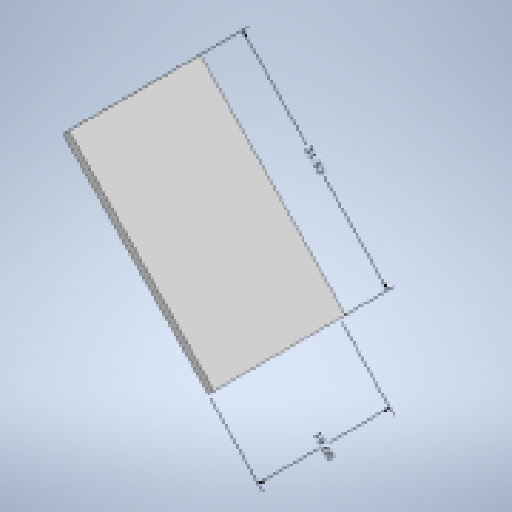
# Autodesk Inventor part: BarraInclinada
Saved by Autodesk Inventor 2024 (Build 280153000, 153)
## iProperties
Created: 2023-07-05
Part Number: BarraInclinada
Material: Genérico
Document SubType Name: Modeling
Designer: sergi
Density: 1 g/cm^3
Appearance: Valor por defecto
Author: sergi
Autodesk Inventor part; units mm, degrees
ref_plane "YZ Plane" through (0, 0, 0) normal (1, 0, 0) x (0, 1, 0)
ref_plane "XZ Plane" through (0, 0, 0) normal (0, 1, 0) x (-1, 0, 0)
ref_plane "XY Plane" through (0, 0, 0) normal (0, 0, 1) x (1, 0, 0)
ref_plane "Plano de trabajo1" through (-734, 252.5, -55) normal (0, 0, -1) x (0, -1, 0)
ref_plane "Plano de trabajo2" through (-30, -30, 770) normal (-1, 0, 0) x (0, 1, 0)
sketch "Boceto4" plane through (-30, -30, 770) normal (-1, 0, 0) x (0, 1, 0)
  line L0 (30, 770) -> (551, 770) projected
  line L1 (1956, 770) -> (581, 770) projected
  line L2 (611, 770) -> (581, 770) projected
  line L3 (30, 770) -> (596, 770)
  line L4 (596, 770) -> (596, 270)
  line L5 (596, 270) -> (30, 270)
  line L6 (30, 270) -> (30, 770)
  dimension "d18" = 566
  dimension "d19" = 500
  constraints: 8 end point, 2 parallel, 1 horizontal, 1 perpendicular
  measures "d18" distance of L4.end L5.end
  measures "d19" distance of L3.end L4.end
extrude "Extrusión4" add sketch "Boceto4" against normal blind 30
